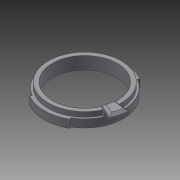
# Autodesk Inventor part: ring
Saved by Autodesk Inventor 2018 (Build 220112000, 112)
## iProperties
Created: 2019-02-20
Part Number: ring
Material: 一般
Document SubType Name: Modeling
Designer: ku_sk
Density: 1 g/cm^3
Appearance: 既定
Author: ku_sk
Autodesk Inventor part; units mm, degrees
ref_plane "YZ Plane" through (0, 0, 0) normal (1, 0, 0) x (0, 1, 0)
ref_plane "XZ Plane" through (0, 0, 0) normal (0, 1, 0) x (-1, 0, 0)
ref_plane "XY Plane" through (0, 0, 0) normal (0, 0, 1) x (1, 0, 0)
sketch "スケッチ1" plane through (0, 0, 0) normal (0, 0, 1) x (1, 0, 0)
  circle A0 centre (0, 0) radius 25.25
  circle A1 centre (0, 0) radius 20.25
  dimension "d0" = 5
  dimension "d1" = 40.5
  constraints: 2 centre point, 2 coincident
  measures "d0" radial gap between concentric circles of A0 A1
  measures "d1" diameter of A1
extrude "押し出し1" add sketch "スケッチ1" along normal blind 8
sketch "スケッチ2" plane through (0, 0, 0) normal (0, 0, 1) x (1, 0, 0)
  circle A0 centre (0, 0) radius 25.25 projected
  arc A1 (8.2256, -22.5996) -> (8.2256, 22.5996) centre (0, 0) ccw
  line L0 (0, -35.35) -> (0, 35.35) projected
  line L1 (8.2256, 22.5996) -> (8.636, 23.7272)
  line L2 (8.2256, -22.5996) -> (8.636, -23.7272)
  line L3 (-35.35, 0) -> (35.35, 0) projected
  point P0 (24.05, 0)
  dimension "d4" = 1.2
  dimension "d5" = 140
  constraints: 5 point on circle, 4 end point, 2 line through centre, 1 centre point, 1 concentric, 1 point on line
  measures "d4" distance of L1.start L1.end
  measures "d5" angle of L2 L1
extrude "押し出し2" cut sketch "スケッチ2" along normal blind 5 contours L3 A1 L1 A0 | A0 L2 A1 L3
mirror "ミラー1" about plane through (0, 0, 0) normal (1, 0, 0) of "押し出し2"
sketch "スケッチ4" plane through (0, 0, 8) normal (0, 0, 1) x (1, 0, 0)
  circle A0 centre (0, 0) radius 25.25 projected
  line L0 (21.7123, -12.5356) -> (0, 0)
  line L1 (-35.8782, 0) -> (38.5193, 0) projected
  arc A1 (23.8972, -19.3516) -> (28.7076, -11.0198) centre (0, 0) ccw
  arc A2 (17.6801, -14.317) -> (21.239, -8.1529) centre (0, 0) ccw
  line L2 (23.8972, -19.3516) -> (17.6801, -14.317)
  line L3 (21.239, -8.1529) -> (28.7076, -11.0198)
  circle A3 centre (0, 0) radius 20.25 projected
  point P0 (26.6303, -15.375)
  point P1 (19.7021, -11.375)
  dimension "d18" = 30
  dimension "d46" = 2.5
  dimension "d47" = 8
  dimension "d48" = 18
  constraints: 6 end point, 6 point on circle, 2 centre point, 2 concentric, 2 line through centre, 2 point on line
  measures "d18" angle of L1 L0
  measures "d46" radial gap between concentric circles of A3 A2
  measures "d47" radial gap between concentric circles of A2 A1
  measures "d48" angle of L3 L2
extrude "押し出し7" add sketch "スケッチ4" along normal blind 2.5 and the other way blind 1 contours L3 A1 L2 A0 | A0 L2 A2 L3
chamfer "面取り4" distance 2.5 angle 45 1 edges at (19.7021, -11.375, 8)
sketch "スケッチ7" plane through (0, 0, 8) normal (0, 0, 1) x (1, 0, 0)
  arc A0 (23.7272, -8.636) -> (19.3426, -16.2304) centre (0, 0) ccw
  arc A1 (21.472, -7.8152) -> (17.5041, -14.6877) centre (0, 0) ccw
  arc A2 (18.905, -7.257) -> (15.7372, -12.7437) centre (0, 0) ccw projected
  line L0 (21.472, -7.8152) -> (23.7272, -8.636)
  arc A3 (23.5729, -9.0488) -> (19.6229, -15.8903) centre (0, 0) ccw projected
  line L1 (17.5041, -14.6877) -> (19.3426, -16.2304)
  line L2 (17.6801, -14.317) -> (23.8972, -19.3516) projected
  line L3 (28.7076, -11.0198) -> (21.239, -8.1529) projected
  dimension "d57" = 1
  dimension "d59" = 2.4
  dimension "d65" = 1
  constraints: 6 point on circle, 4 end point, 3 line through centre, 2 centre point, 2 concentric
  measures "d57" angle of L2 L1
  measures "d59" distance of L1.start L1.end
  measures "d65" angle of L3 L0
extrude "押し出し8" cut sketch "スケッチ7" against normal blind 3
chamfer "面取り5" distance 1.5 angle 45 5 edges at (26.6303, -15.375, 10.5) (21.239, -8.1529, 10.5) (24.9733, -9.5863, 10.5) (17.6801, -14.317, 10.5) (20.7887, -16.8343, 10.5)
